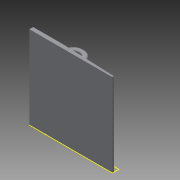
# Autodesk Inventor part: ESP_DISP_LG
Saved by Autodesk Inventor 2015 (Build 190159000, 159)
## iProperties
Created: 2018-04-04
Part Number: ESP_DISP_LG
Material: Типовые
Document SubType Name: Modeling
Designer: JOK
Density: 1 g/cm^3
Appearance: По умолчанию
Author: JOK
Autodesk Inventor part; units mm, degrees
ref_plane "YZ Plane" through (0, 0, 0) normal (1, 0, 0) x (0, 1, 0)
ref_plane "XZ Plane" through (0, 0, 0) normal (0, 1, 0) x (-1, 0, 0)
ref_plane "XY Plane" through (0, 0, 0) normal (0, 0, 1) x (1, 0, 0)
sketch "Эскиз1" plane through (0, 0, 0) normal (0, 1, 0) x (-1, 0, 0)
  line L0 (3.5, 13) -> (-3.5, 13)
  line L1 (-3.5, 13) -> (-3.5, 3)
  line L2 (-3.5, 3) -> (3.5, 3)
  line L3 (3.5, 3) -> (3.5, 13)
  line L4 (3.5, 13) -> (-3.5, 3) construction
  line L5 (-3.5, 13) -> (3.5, 3) construction
  line L6 (5, 21) -> (-5, 21)
  line L7 (-5, 21) -> (-5, -5)
  line L8 (-5, -5) -> (5, -5)
  line L9 (5, -5) -> (5, 21)
  line L10 (5, 21) -> (-5, -5) construction
  line L11 (-5, 21) -> (5, -5) construction
  point P0 (0, 0)
  point P1 (0, 8)
  point P2 (0, 8)
  dimension "d0" = 7
  dimension "d1" = 10
  constraints: 24 end point, 5 midpoint, 4 parallel, 2 horizontal, 2 perpendicular
  measures "d0" distance of L2.end L1.end
  measures "d1" distance of L1.end L0.end
extrude "Выдавливание1" add sketch "Эскиз1" along normal blind 2 contours L3 L2 L1 L0 | L9 L8 L7 L6
sketch "Эскиз2" plane through (0, 2, 0) normal (0, 1, 0) x (1, 0, 0)
  line L0 (-5, -21) -> (5, -21) projected
  line L1 (5, -21) -> (5, 5) projected
  line L2 (5, 5) -> (-5, 5) projected
  line L3 (-5, 5) -> (-5, -21) projected
  point P0 (0, 0)
chamfer "Фаска1" distance 1.4 angle 30 4 edges at (0, 2, 21) (5, 2, 8) (0, 2, -5) (-5, 2, 8) measured on face at (1.6667, 2, 12.3333)
sketch "Эскиз3" plane through (0, 2, 0) normal (0, 1, 0) x (1, 0, 0)
  line L0 (-3.25, -12.0714) -> (3.25, -12.0714)
  line L1 (3.25, -12.0714) -> (3.25, -2.7857)
  line L2 (3.25, -2.7857) -> (-3.25, -2.7857)
  line L3 (-3.25, -2.7857) -> (-3.25, -12.0714)
  line L4 (-3.25, -12.0714) -> (3.25, -2.7857) construction
  line L5 (3.25, -12.0714) -> (-3.25, -2.7857) construction
  point P0 (0, 0)
  point P1 (0, -7.4286)
  dimension "d7" = 6.5
  constraints: 12 end point, 2 midpoint, 2 parallel, 1 horizontal, 1 perpendicular
  measures "d7" distance of L2.end L1.end
extrude "Выдавливание2" add sketch "Эскиз3" along normal blind 10
fillet "Сопряжение1" radius 3 2 edges at (3.25, 12, 7.4286) (-3.25, 12, 7.4286)
sketch "Эскиз4" plane through (3.25, 2, 2.7857) normal (0, 0, -1) x (-1, 0, 0)
  line L0 (3, 10) -> (3.5, 10) projected
  line L1 (3.25, 10) -> (3.25, 7)
  circle A0 centre (3.25, 7) radius 1.75
  point P0 (3.25, -2)
  dimension "d11" = 3
  dimension "d12" = 3.5
  constraints: 2 end point, 1 centre point, 1 coincident, 1 midpoint, 1 vertical
  measures "d11" distance of L1.start L1.end
  measures "d12" diameter of A0
extrude "Выдавливание3" cut sketch "Эскиз4" against normal blind 10
fillet "Сопряжение2" radius 0.4 2 edges at (1.75, 9, 2.7857) (1.75, 9, 12.0714)
fillet "Сопряжение3" radius 0.4 10 edges at (3.25, 5.5, 12.0714) (0, 12, 12.0714) (-2.3713, 11.1213, 12.0714) (-3.25, 5.5, 12.0714) (2.3713, 11.1213, 12.0714) (0, 12, 2.7857) (-2.3713, 11.1213, 2.7857) (-3.25, 5.5, 2.7857) (3.25, 5.5, 2.7857) (2.3713, 11.1213, 2.7857)
sketch "Эскиз5" plane through (0, 0, 0) normal (0, -1, 0) x (1, 0, 0)
  line L0 (-5, 21) -> (5, 21) projected
  line L1 (-5, -5) -> (-5, 21) projected
  line L2 (5, -5) -> (-5, -5) projected
  line L3 (5, 21) -> (5, -5) projected
  line L4 (-5, 21) -> (21, 21)
  line L5 (21, 21) -> (21, -5)
  line L6 (21, -5) -> (-5, -5)
  line L7 (-5, -5) -> (-5, 21)
  point P0 (0, 0)
  constraints: 8 end point, 2 parallel, 1 horizontal, 1 perpendicular
extrude "Выдавливание4" add sketch "Эскиз5" against normal blind 2 contours L4 L5 L6 L3
sketch "Эскиз6" plane through (-5, 0, -5) normal (0, 0, -1) x (-1, 0, 0)
  line L0 (-10, 1.1917) -> (0, 1.1917) projected
  line L1 (-10, 1.1917) -> (-10, 2) projected
  line L2 (-26, 2) -> (-10, 2) projected
  line L3 (-26, 0) -> (-26, 2) projected
  line L4 (0, 0) -> (-26, 0) projected
  line L5 (0, 0) -> (0, 1.1917) projected
  point P0 (-5, 0)
sketch "Эскиз7" plane through (-5, 0, -5) normal (0, 0, -1) x (-1, 0, 0)
  line L0 (-10, 1.1917) -> (0, 1.1917) projected
  line L1 (-10, 1.1917) -> (-10, 2) projected
  line L2 (0, 0) -> (-26, 0) projected
  line L3 (0, 0) -> (0, 1.1917) projected
  line L4 (-10, 2) -> (-26, 2)
  line L5 (-26, 2) -> (-26, 0.5)
  line L6 (-26, 0) -> (-10, 0)
  line L7 (-10, 0) -> (-10, 1.1917)
  line L8 (-26, 1) -> (-26, 0)
  line L9 (-10, 1.1917) -> (-26, 0.5)
  line L10 (-26, 0.5) -> (-26, 0)
  line L11 (-10, 1.1917) -> (-10, 2)
  line L12 (-10, 1.1917) -> (-10, 2)
  line L13 (-10, 0) -> (-10, 1.1917)
  point P0 (-5, 0)
  constraints: 20 end point, 5 parallel, 3 collinear, 2 perpendicular, 1 horizontal, 1 midpoint, 1 vertical
extrude "Выдавливание5" cut sketch "Эскиз7" against normal blind 26 contours L9 L5 L4 L1
